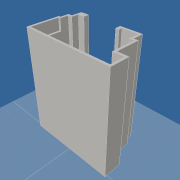
# Autodesk Inventor part: Gehäuse
Saved by Autodesk Inventor 2016 SP2 (Build 200236200, 236)
## iProperties
Created: 2018-07-08
Part Number: Gehäuse
Material: Generisch
Document SubType Name: Modeling
Designer: User
Density: 1 g/cm^3
Appearance: Vorgabe
Author: User
Autodesk Inventor part; units mm, degrees
ref_plane "YZ Plane" through (0, 0, 0) normal (1, 0, 0) x (0, 1, 0)
ref_plane "XZ Plane" through (0, 0, 0) normal (0, 1, 0) x (-1, 0, 0)
ref_plane "XY Plane" through (0, 0, 0) normal (0, 0, 1) x (1, 0, 0)
sketch "Skizze1" plane through (0, 0, 0) normal (0, 0, 1) x (1, 0, 0)
  line L0 (-60, 0) -> (60, 0)
  line L1 (60, 0) -> (60, 20)
  line L2 (60, 20) -> (45, 20)
  line L3 (45, 20) -> (45, 54)
  line L4 (38.5, 70) -> (-50.5, 70)
  line L5 (-60, 41) -> (-60, 0)
  line L6 (-60, 57) -> (-60, 44)
  line L7 (-60, 44) -> (-63, 44)
  line L8 (-63, 44) -> (-63, -3)
  line L9 (-63, -3) -> (63, -3)
  line L10 (63, -3) -> (63, 23)
  line L11 (63, 23) -> (48, 23)
  line L12 (48, 23) -> (48, 57)
  line L13 (41.5, 73) -> (-53.5, 73)
  line L14 (-60, 41) -> (-57, 41)
  line L15 (-57, 54) -> (-50.5, 54)
  line L16 (-50.5, 54) -> (-50.5, 70)
  line L17 (-60, 57) -> (-53.5, 57)
  line L18 (-53.5, 73) -> (-53.5, 57)
  line L19 (-57, 54) -> (-57, 41)
  line L20 (-50.5, 70) -> (-40.5, 70)
  line L21 (-40.5, 70) -> (-40.5, 65)
  line L22 (-40.5, 65) -> (-50.5, 65)
  line L23 (-50.5, 65) -> (-50.5, 70)
  line L24 (10.5, 70) -> (15.5, 70)
  line L25 (15.5, 70) -> (15.5, 65)
  line L26 (15.5, 65) -> (10.5, 65)
  line L27 (10.5, 65) -> (10.5, 70)
  line L28 (41.5, 73) -> (41.5, 57)
  line L29 (41.5, 57) -> (48, 57)
  line L30 (38.5, 70) -> (38.5, 54)
  line L31 (38.5, 54) -> (45, 54)
  line L32 (-60, 0) -> (-52, 0)
  line L33 (-52, 0) -> (-52, 6)
  line L34 (-52, 6) -> (-60, 6)
  line L35 (-60, 6) -> (-60, 0)
  line L36 (24.5, 6) -> (31.5, 6)
  line L37 (31.5, 6) -> (31.5, 0)
  line L38 (31.5, 0) -> (24.5, 0)
  line L39 (24.5, 0) -> (24.5, 6)
  line L40 (-57, 41) -> (-60, 41)
  line L41 (-60, 41) -> (-60, 6)
  line L42 (-60, 6) -> (-57, 6)
  line L43 (-57, 6) -> (-57, 41)
  line L44 (-50.5, 59.5) -> (38.5, 59.5)
  line L45 (-50.5, 59.5) -> (-50.5, 65)
  line L46 (-50.5, 65) -> (-40.5, 65)
  line L47 (-40.5, 65) -> (-40.5, 70)
  line L48 (-40.5, 70) -> (10.5, 70)
  line L49 (10.5, 70) -> (10.5, 65)
  line L50 (10.5, 65) -> (15.5, 65)
  line L51 (15.5, 65) -> (15.5, 70)
  line L52 (15.5, 70) -> (38.5, 70)
  line L53 (38.5, 70) -> (38.5, 59.5)
  point P0 (0, 0)
  point P1 (41.5, 70)
  point P2 (0, 0)
  dimension "d0" = 120
  dimension "d9" = 15
  dimension "d13" = 70
  dimension "d17" = 3
  dimension "d18" = 3
  dimension "d19" = 3
  dimension "d20" = 3
  dimension "d30" = 3
  dimension "d31" = 20
  dimension "d32" = 41
  dimension "d37" = 3
  dimension "d38" = 54
  dimension "d39" = 3
  dimension "d41" = 3
  dimension "d43" = 3
  dimension "d47" = 10
  dimension "d48" = 5
  dimension "d49" = 51
  dimension "d50" = 3
  dimension "d51" = 3
  dimension "d52" = 89
  dimension "d53" = 8
  dimension "d54" = 6
  dimension "d55" = 8
  dimension "d58" = 3
  dimension "d59" = 3
  dimension "d60" = 7
  dimension "d61" = 76.5
  dimension "d68" = 5.5
  constraints: 109 end point, 28 perpendicular, 10 parallel, 8 horizontal, 7 collinear, 5 point on line, 2 vertical, 1 coincident, 1 midpoint
  measures "d0" distance between parallel lines of L1 L5
  measures "d9" distance between parallel lines of L1 L3
  measures "d13" distance between parallel lines of L0 L4
  measures "d17" distance between parallel lines of L9 L0
  measures "d18" distance between parallel lines of L10 L1
  measures "d19" distance between parallel lines of L12 L3
  measures "d20" distance between parallel lines of L2 L11
  measures "d30" distance between parallel lines of L14 L7
  measures "d31" distance between parallel lines of L0 L2
  measures "d32" distance between parallel lines of L0 L14
  measures "d37" distance between parallel lines of L15 L17
  measures "d38" distance between parallel lines of L0 L15
  measures "d39" distance between parallel lines of L19 L6
  measures "d41" distance between parallel lines of L16 L18
  measures "d43" distance between parallel lines of L4 L13
  measures "d47" distance of L21.end L22.end
  measures "d48" distance of L25.end L26.end
  measures "d49" distance between parallel lines of L27 L21
  measures "d50" distance between parallel lines of L28 L30
  measures "d51" distance between parallel lines of L31 L29
  measures "d52" distance between parallel lines of L30 L16
  measures "d53" distance between parallel lines of L22 L13
  measures "d54" distance of L32.end L33.end
  measures "d55" distance of L33.end L34.end
  measures "d58" distance between parallel lines of L5 L8
  measures "d59" distance between parallel lines of L6 L8
  measures "d60" distance of L36.start L36.end
  measures "d61" distance between parallel lines of L39 L33
  measures "d68" distance between parallel lines of L44 L22
extrude "Extrusion1" add sketch "Skizze1" along normal blind 150 contours L16 L4 L21 L22 | L25 L26 L27 L4 | L17 L18 L13 L28 L29 L12 L11 L10 L9 L8 L7 L6
extrude "Extrusion3" add sketch "Skizze1" along normal blind 133 contours L5 L34 L33 L0 | L5 L14 L43 L34
sketch "Skizze3" plane through (-53.5, 73, 0) normal (0, 1, 0) x (1, 0, 0)
  line L0 (13, -62) -> (64, -62)
  line L1 (64, -62) -> (64, -150)
  line L2 (64, -150) -> (13, -150)
  line L3 (13, -150) -> (13, -62)
  line L4 (0, 0) -> (0, -150) projected
  line L5 (95, -150) -> (0, -150) projected
  point P0 (60, 0)
  dimension "d25" = 51
  dimension "d26" = 88
  dimension "d45" = 13
  constraints: 8 end point, 2 parallel, 1 collinear, 1 horizontal, 1 perpendicular
  measures "d25" distance between parallel lines of L1 L3
  measures "d26" distance of L2.end L0.start
  measures "d45" distance between parallel lines of L3 L4
extrude "Extrusion2" cut sketch "Skizze3" against normal up to surface (3 mm away)
extrude "Extrusion5" add sketch "Skizze1" along normal blind 55 contours L16 L22 L21 L4 L27 L26 L25 L30 L44
equation "\"d18\" = d20"
equation "\"d19\" = d20"
equation "\"d30\" = d20"
equation "\"d37\" = d20"
equation "\"d39\" = d20"
equation "\"d41\" = d20"
equation "\"d43\" = d20"
equation "\"d50\" = d20"
equation "\"d51\" = d20"
equation "\"d58\" = d20"
